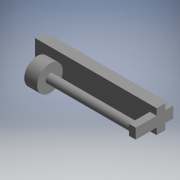
# Autodesk Inventor part: 3385160 HGPL-BAC-14-40---(J)
Saved by Autodesk Inventor 2017.3 (Build 213256000, 256)
## iProperties
Part Number: 3385160 HGPL-BAC-14-40---(J)
Material: Generic
Catalog Web Link: www.cadenas.de
Description: HGPL-B-(J)-gripping jaw
Vendor: FESTO
Document SubType Name: Modeling
Designer: partserver
Manufacturer: FESTO
Mass: 9.46808 g
Surface Area: 54.3996 cm^2
Volume: 9.46808 cm^3
Density: 1 g/cm^3
Appearance: PSOLRGB-175-175-175
Category: PARTsolutions
Company: FESTO
Title: 3385160 HGPL-BAC-14-40
Author: Cadenas PARTsolutions
Comments: gripping jaw
PSOL_IDENT_0: {$CADENAS_DATA\23d-libs\festo\parts\h\hgpl\hgpl_b\parts\hgpl_b_jaw.prj},194 {VTYP=3D},{NB=3385160 HG
PSOL_IDENT_1: PL-BAC-14-40---(J)},{LINA=3385160 HGPL-BAC-14-40},{NN=HGPL-B-(J)},{DATE=11.03.2020 14:57:17},{GEOMDA
PSOL_IDENT_2: TE=08.01.2020 15:11:00},{VERSION=},{LINEID=10},{WBVAR=},{WBNUMERIC=}  {NB=3385160 HGPL-BAC-14-40---(
PSOL_IDENT_3: J)},{LINA=3385160 HGPL-BAC-14-40},{KT=DUMMY},{TNR=3385160},{TYP=HGPL-BAC-14-40},{HUB=40.000},{KDM=14
PSOL_IDENT_4: },{BACKEN=14-40},{B1=13.600},{B2=6.500},{B22=6.000},{L1=67.100},{L2=4.300},{L3=8.000},{H1=9.800},{H2=
PSOL_IDENT_5: 5.000},{H3=7.000},{D2=5.000},{DG2=3.000},{T3=1.300},{T4=5.500},{H18G=8.800},{L23G=18.000},{L18G=21.0
PSOL_IDENT_6: 00},{L1G=113.600},{R7G=7.500},{SN=4.000}
NB: 3385160 HGPL-BAC-14-40---(J)
NN: HGPL-B-(J)
NT: gripping jaw
NBSYN: $TNR. $TYP.---(J)
LINA: 3385160 HGPL-BAC-14-40
CATALOG: Festo
TNR: 3385160
TYP: HGPL-BAC-14-40
HUB: 40
KDM: 14
B22: 6
L1: 67.1
L2: 4.3
L3: 8
H3: 7
D2: 5
DG2: 3
T3: 1.3
T4: 5.5
H18G: 8.8
L23G: 18
L18G: 21
L1G: 113.6
R7G: 7.5
SN: 4
SUPPLIER: FESTO
ARTICLENO: 3385160 HGPL-BAC-14-40---(J)
BOMINFO: 3385160 HGPL-BAC-14-40
CREATOR: CADENAS GmbH
Autodesk Inventor part; units mm, degrees
sketch "Skizze_1" plane through (-37.55, 0, 0) normal (1, 0, 0) x (0, 0, -1)
  line L0 (-6.8, 5) -> (-6.8, 0)
  line L1 (-6.8, 0) -> (6.8, 0)
  line L2 (6.8, 0) -> (6.8, 5)
  line L3 (6.8, 5) -> (3.25, 5)
  line L4 (3.25, 5) -> (3.25, 9.8)
  line L5 (3.25, 9.8) -> (-3.25, 9.8)
  line L6 (-3.25, 9.8) -> (-3.25, 5)
  line L7 (-3.25, 5) -> (-6.8, 5)
  constraints: 16 end point
extrude "Extrusion1" add sketch "Skizze_1" along normal blind 71.1
sketch "Skizze_2" plane through (0, 0, 0) normal (0, 0, 1) x (1, 0, 0)
  line L0 (-37.55, 7) -> (-37.55, -12.2)
  line L1 (-37.55, -12.2) -> (-33.55, -12.2)
  line L2 (-33.55, -12.2) -> (-33.55, 7)
  line L3 (-33.55, 7) -> (-37.55, 7)
  constraints: 8 end point
extrude "Extrusion2" add sketch "Skizze_2" along normal mid plane 6
sketch "Sketch_1" plane through (0, 0, 0) normal (0, 0, 1) x (1, 0, 0)
  line L0 (23.25, -9.2) -> (-33.55, -9.2)
  line L1 (-33.55, -9.2) -> (-33.55, -6.7)
  line L2 (-33.55, -6.7) -> (15.6767, -6.7)
  line L3 (15.6767, -6.7) -> (15.6767, -1.7)
  line L4 (15.6767, -1.7) -> (23.25, -1.7)
  line L5 (23.25, -1.7) -> (23.25, -9.2)
  line L6 (23.25, -9.2) -> (-33.55, -9.2)
  constraints: 14 end point
revolve "Revolution1" add sketch "Sketch_1" angle 360 about axis through (23.25, -9.2, 0) along (1, 0, 0)
sketch "Sketch_3" plane through (29.25, 0, 0) normal (1, 0, 0) x (0, 0, -1)
  line L0 (0, 9.8) -> (0, 0.6401)
  line L1 (0, 0.6401) -> (-1.2295, 1.35)
  line L2 (-1.2295, 1.35) -> (-1.2295, 8.2295)
  line L3 (-1.2295, 8.2295) -> (-1.5, 8.5)
  line L4 (-1.5, 8.5) -> (-2.5, 8.5)
  line L5 (-2.5, 8.5) -> (-2.5, 9.8)
  line L6 (-2.5, 9.8) -> (0, 9.8)
  line L7 (0, 9.8) -> (0, 0.6401)
  constraints: 16 end point
revolve "Revolution2" cut sketch "Sketch_3" angle 360 about axis through (29.25, 9.8, 0) along (0, 1, 0)
thread "Thread1" size "M3x0.5" class "6H" standard "ISO Metric profile" length 5.2295
pattern_linear "Rectangular Pattern1" count 3 spacing 8 along (-1, 0, 0) of "Revolution2"
ref_plane "ANBAU_XY" through (23.25, -9.2, 0) normal (1, 0, 0) x (0, 0, -1)
ref_plane "ANBAU_YZ" through (23.25, -9.2, 0) normal (0, 0, -1) x (0, 1, 0)
ref_plane "ANBAU_ZX" through (23.25, -9.2, 0) normal (0, 1, 0) x (1, 0, 0)
ref_plane "SCHRAUBE_1_XY" through (29.25, 8.5, 0) normal (0, 1, 0) x (1, 0, 0)
ref_plane "SCHRAUBE_1_YZ" through (29.25, 8.5, 0) normal (1, 0, 0) x (0, 0, -1)
ref_plane "SCHRAUBE_1_ZX" through (29.25, 8.5, 0) normal (0, 0, -1) x (0, 1, 0)
ref_plane "SCHRAUBE_2_XY" through (21.25, 8.5, 0) normal (0, 1, 0) x (1, 0, 0)
ref_plane "SCHRAUBE_2_YZ" through (21.25, 8.5, 0) normal (1, 0, 0) x (0, 0, -1)
ref_plane "SCHRAUBE_2_ZX" through (21.25, 8.5, 0) normal (0, 0, -1) x (0, 1, 0)
ref_plane "SCHRAUBE_3_XY" through (13.25, 8.5, 0) normal (0, 1, 0) x (1, 0, 0)
ref_plane "SCHRAUBE_3_YZ" through (13.25, 8.5, 0) normal (1, 0, 0) x (0, 0, -1)
ref_plane "SCHRAUBE_3_ZX" through (13.25, 8.5, 0) normal (0, 0, -1) x (0, 1, 0)
ref_plane "ZBHJAW1_XY" through (29.25, 8.5, 0) normal (0, -1, 0) x (1, 0, 0)
ref_plane "ZBHJAW1_YZ" through (29.25, 8.5, 0) normal (1, 0, 0) x (0, 0, 1)
ref_plane "ZBHJAW1_ZX" through (29.25, 8.5, 0) normal (0, 0, 1) x (0, -1, 0)
ref_plane "ZBHJAW2_XY" through (13.25, 8.5, 0) normal (0, -1, 0) x (1, 0, 0)
ref_plane "ZBHJAW2_YZ" through (13.25, 8.5, 0) normal (1, 0, 0) x (0, 0, 1)
ref_plane "ZBHJAW2_ZX" through (13.25, 8.5, 0) normal (0, 0, 1) x (0, -1, 0)
body "Solid1"
